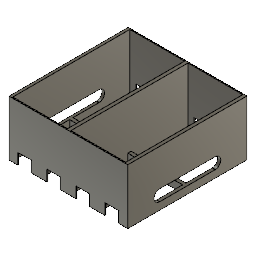
Jar Holder (Autodesk Fusion 360 design; units mm, degrees)
Autodesk Fusion 360 part; units mm, degrees
sketch "Schizzo1" plane through (0, 0, 0) normal (0, 0, 1) x (1, 0, 0)
  line L0 (0, 0) -> (214.4, 0)
  line L1 (214.4, 0) -> (214.4, 215)
  line L2 (214.4, 215) -> (0, 215)
  line L3 (0, 215) -> (0, 0)
  line L4 (51.4, 0) -> (5, 0)
  line L5 (57.4, 104.5) -> (103.8, 104.5)
  line L6 (57.4, 2) -> (57.4, 104.5)
  line L7 (103.8, 104.5) -> (103.8, 2)
  line L8 (109.8, 104.5) -> (156.2, 104.5)
  line L9 (109.8, 2) -> (109.8, 104.5)
  line L10 (156.2, 104.5) -> (156.2, 2)
  line L11 (162.2, 2) -> (162.2, 104.5)
  line L12 (162.2, 104.5) -> (208.6, 104.5)
  line L13 (208.6, 104.5) -> (208.6, 2)
  line L14 (5, 110.5) -> (5, 213)
  line L15 (5, 213) -> (51.4, 213)
  line L16 (51.4, 213) -> (51.4, 110.5)
  line L17 (57.4, 110.5) -> (57.4, 213)
  line L18 (57.4, 213) -> (103.8, 213)
  line L19 (103.8, 213) -> (103.8, 110.5)
  line L20 (109.8, 110.5) -> (109.8, 213)
  line L21 (109.8, 213) -> (156.2, 213)
  line L22 (156.2, 213) -> (156.2, 110.5)
  line L23 (162.2, 110.5) -> (162.2, 213)
  line L24 (162.2, 213) -> (208.6, 213)
  line L25 (208.6, 213) -> (208.6, 110.5)
  line L26 (5, 110.5) -> (51.4, 110.5)
  line L27 (103.8, 110.5) -> (57.4, 110.5)
  line L28 (109.8, 110.5) -> (156.2, 110.5)
  line L29 (208.6, 110.5) -> (162.2, 110.5)
  line L30 (57.4, 2) -> (103.8, 2)
  line L31 (156.2, 2) -> (109.8, 2)
  line L32 (162.2, 2) -> (208.6, 2)
  line L33 (5, 104.5) -> (51.4, 104.5)
  line L34 (51.4, 104.5) -> (51.4, 2)
  line L35 (51.4, 2) -> (5, 2)
  line L36 (5, 2) -> (5, 104.5)
  line L37 (5, 110.5) -> (5, 104.5)
  line L38 (51.4, 110.5) -> (51.4, 104.5)
  line L39 (51.4, 104.5) -> (57.4, 104.5)
  line L40 (51.4, 110.5) -> (57.4, 110.5)
  line L41 (103.8, 110.5) -> (109.8, 110.5)
  line L42 (103.8, 104.5) -> (109.8, 104.5)
  line L43 (103.8, 110.5) -> (103.8, 104.5)
  line L44 (109.8, 110.5) -> (109.8, 104.5)
  line L45 (57.4, 110.5) -> (57.4, 104.5)
  line L46 (156.2, 110.5) -> (156.2, 104.5)
  line L47 (162.2, 110.5) -> (162.2, 104.5)
  line L48 (156.2, 110.5) -> (162.2, 110.5)
  line L49 (156.2, 104.5) -> (5.3108, 104.5)
  line L50 (4.8606, 104.5) -> (-21.6126, 104.5)
  line L51 (-21.6126, 104.5) -> (-37.5505, 104.5)
  line L52 (5, 213) -> (5, 215)
  line L53 (5, 2) -> (5, 0)
  line L54 (208.6, 2) -> (208.6, 0)
  line L55 (162.2, 104.5) -> (156.2, 104.5)
  line L56 (208.6, 213) -> (208.6, 215)
  line L57 (208.6, 110.5) -> (208.6, 104.5)
  line L58 (80.6, 2) -> (80.6, 0)
  line L59 (133, 2) -> (133, 0)
  line L60 (80.6, 213) -> (80.6, 215)
  line L61 (133, 213) -> (133, 215)
  line L62 (5, 2) -> (0, 2)
  line L63 (51.4, 2) -> (57.4, 2)
  line L64 (103.8, 2) -> (109.8, 2)
  line L65 (156.2, 2) -> (162.2, 2)
  line L66 (208.6, 2) -> (214.4, 2)
  line L67 (208.6, 213) -> (214.4, 213)
  line L68 (156.2, 213) -> (162.2, 213)
  line L69 (103.8, 213) -> (109.8, 213)
  line L70 (51.4, 213) -> (57.4, 213)
  line L71 (0, 213) -> (5, 213)
  dimension "d1" = 214.4
  dimension "d2" = 215
  dimension "d6" = 46.4
  dimension "d7" = 102.5
  dimension "d8" = 46.4
  dimension "d9" = 102.5
  dimension "d10" = 46.4
  dimension "d11" = 102.5
  dimension "d13" = 6
  dimension "d14" = 6
  dimension "d15" = 46.4
  dimension "d16" = 102.5
  dimension "d17" = 46.4
  dimension "d19" = 46.4
  dimension "d20" = 102.5
  dimension "d21" = 46.4
  dimension "d22" = 102.5
  dimension "d23" = 6
  dimension "d24" = 6
  dimension "d25" = 6
  dimension "d26" = 46.4
  dimension "d27" = 102.5
  dimension "d28" = 6
  dimension "d29" = 6
  constraint horizontal L0
  constraint vertical L1
  constraint horizontal L2
  constraint vertical L3
  constraint coincident L0.start L3.end
  constraint horizontal L4
  constraint collinear L0 L4
  constraint horizontal L5
  constraint vertical L7
  constraint vertical L6
  constraint horizontal L8
  constraint vertical L10
  constraint vertical L9
  constraint horizontal L12
  constraint vertical L13
  constraint vertical L11
  constraint horizontal L15
  constraint vertical L16
  constraint vertical L14
  constraint horizontal L18
  constraint vertical L19
  constraint vertical L17
  constraint horizontal L21
  constraint vertical L22
  constraint vertical L20
  constraint horizontal L24
  constraint vertical L25
  constraint vertical L23
  constraint perpendicular L16 L26
  constraint perpendicular L17 L27
  constraint perpendicular L22 L28
  constraint perpendicular L23 L29
  constraint perpendicular L7 L30
  constraint perpendicular L9 L31
  constraint perpendicular L13 L32
  constraint horizontal L33
  constraint vertical L34
  constraint horizontal L35
  constraint vertical L36
  constraint perpendicular L33 L37
  constraint perpendicular L6 L39
  constraint perpendicular L17 L40
  constraint perpendicular L20 L41
  constraint perpendicular L9 L42
  constraint perpendicular L47 L48
  constraint perpendicular L14 L49
  constraint perpendicular L14 L50
  constraint perpendicular L14 L51
  constraint coincident L2 L52.end
  constraint perpendicular L2 L52
  constraint perpendicular L35 L53
  constraint coincident L0 L54.end
  constraint perpendicular L0 L54
  constraint perpendicular L46 L55
  constraint coincident L2 L56.end
  constraint perpendicular L2 L56
  constraint midpoint L30 L58.start
  constraint coincident L0 L58.end
  constraint perpendicular L0 L58
  constraint midpoint L31 L59.start
  constraint coincident L0 L59.end
  constraint perpendicular L0 L59
  constraint midpoint L18 L60.start
  constraint coincident L2 L60.end
  constraint perpendicular L2 L60
  constraint midpoint L21 L61.start
  constraint coincident L2 L61.end
  constraint perpendicular L2 L61
  constraint coincident L3 L62.end
  constraint perpendicular L3 L62
  constraint coincident L1 L66.end
  constraint perpendicular L1 L66
  constraint coincident L1 L67.end
  constraint perpendicular L1 L67
  constraint perpendicular L20 L69
  constraint coincident L3 L71.start
  constraint perpendicular L14 L71
  measures "d1" distance of L0.start L0.end
  measures "d2" distance of L0.start L2.end
  measures "d6" distance of L5.start L5.end
  measures "d7" distance of L6.start L5.start
  measures "d8" distance of L8.start L8.end
  measures "d9" distance of L8.start L9.start
  measures "d10" distance of L11.end L12.end
  measures "d11" distance of L11.end L11.start
  measures "d13" distance of L7 L9
  measures "d14" distance of L10 L11
  measures "d15" distance of L14.end L15.end
  measures "d16" distance of L14.start L14.end
  measures "d17" distance of L17.end L18.end
  measures "d19" distance of L20.end L21.end
  measures "d20" distance of L20.end L20.start
  measures "d21" distance of L23.end L24.end
  measures "d22" distance of L23.end L23.start
  measures "d23" distance of L16 L17
  measures "d24" distance of L19 L20
  measures "d25" distance of L22 L23
  measures "d26" distance of L33.start L33.end
  measures "d27" distance of L33.start L35.end
  measures "d28" distance of L6 L34
  measures "d29" distance of L26 L33
extrude "Estrusione1" add sketch "Schizzo1" along normal blind 100 contours L0 L3 L53 L62 | L0 L4 L30 L35 L53 L58 L63 | L3 L14 L36 L37 L62 L71 | L0 L30 L31 L58 L59 L64 | L6 L34 L39 L49 L63 | L26 L33 L37 L38 L49 | L2 L3 L52 L71 | L0 L31 L32 L54 L59 L65 | L38 L39 L40 L45 L49 | L2 L15 L18 L52 L60 L70 | L0 L1 L54 L66 | L7 L9 L42 L49 L64 | L16 L17 L40 L70 | L5 L27 L43 L45 L49 | L1 L13 L25 L57 L66 L67 | L10 L11 L55 L65 | L41 L42 L43 L44 L49 | L2 L18 L21 L60 L61 L69 | L12 L29 L47 L57 | L8 L28 L44 L46 L49 | L46 L47 L48 L55 | L19 L20 L41 L69 | L2 L21 L24 L56 L61 L68 | L1 L2 L56 L67 | L22 L23 L48 L68 makes body 1
sketch "Schizzo2" plane through (0, 0, 0) normal (0, 0, 1) x (1, 0, 0)
  line L0 (16, 222.0493) -> (40.4, 222.0493)
  line L1 (40.4, 222.0493) -> (40.4, 197.6493)
  line L2 (40.4, 197.6493) -> (16, 197.6493)
  line L3 (16, 197.6493) -> (16, 222.0493)
  line L4 (5, 110.5) -> (5, 213)
  line L5 (68.4, 222.0493) -> (92.8, 222.0493)
  line L6 (92.8, 222.0493) -> (92.8, 197.6493)
  line L7 (68.4, 197.6493) -> (68.4, 222.0493)
  line L8 (92.8, 197.6493) -> (68.4, 197.6493)
  line L9 (120.8, 197.6493) -> (120.8, 222.0493)
  line L10 (145.2, 197.6493) -> (120.8, 197.6493)
  line L11 (145.2, 222.0493) -> (145.2, 197.6493)
  line L12 (120.8, 222.0493) -> (145.2, 222.0493)
  line L13 (173.2, 222.0493) -> (197.6, 222.0493)
  line L14 (173.2, 197.6493) -> (173.2, 222.0493)
  line L15 (197.6, 197.6493) -> (173.2, 197.6493)
  line L16 (197.6, 222.0493) -> (197.6, 197.6493)
  line L17 (92.8, -12.3507) -> (68.4, -12.3507)
  line L18 (16, 12.0493) -> (40.4, 12.0493)
  line L19 (16, -12.3507) -> (16, 12.0493)
  line L20 (40.4, -12.3507) -> (16, -12.3507)
  line L21 (40.4, 12.0493) -> (40.4, -12.3507)
  line L22 (68.4, -12.3507) -> (68.4, 12.0493)
  line L23 (68.4, 12.0493) -> (92.8, 12.0493)
  line L24 (92.8, 12.0493) -> (92.8, -12.3507)
  line L25 (120.8, -12.3507) -> (120.8, 12.0493)
  line L26 (120.8, 12.0493) -> (145.2, 12.0493)
  line L27 (145.2, -12.3507) -> (120.8, -12.3507)
  line L28 (145.2, 12.0493) -> (145.2, -12.3507)
  line L29 (173.2, -12.3507) -> (173.2, 12.0493)
  line L30 (173.2, 12.0493) -> (197.6, 12.0493)
  line L31 (197.6, 12.0493) -> (197.6, -12.3507)
  line L32 (197.6, -12.3507) -> (173.2, -12.3507)
  dimension "d32" = 24.4
  dimension "d33" = 24.4
  dimension "d34" = 11
  dimension "d35" = 24.4
  dimension "d36" = 24.4
  dimension "d37" = 24.4
  dimension "d38" = 24.4
  dimension "d39" = 24.4
  dimension "d40" = 24.4
  dimension "d41" = 24.4
  dimension "d42" = 24.4
  dimension "d43" = 24.4
  dimension "d44" = 24.4
  dimension "d45" = 24.4
  dimension "d46" = 24.4
  dimension "d47" = 24.4
  dimension "d48" = 24.4
  constraint horizontal L0
  constraint vertical L1
  constraint horizontal L2
  constraint vertical L3
  constraint horizontal L5
  constraint vertical L6
  constraint horizontal L8
  constraint vertical L7
  constraint horizontal L12
  constraint vertical L11
  constraint horizontal L10
  constraint vertical L9
  constraint horizontal L13
  constraint vertical L16
  constraint horizontal L15
  constraint vertical L14
  constraint horizontal L18
  constraint vertical L21
  constraint horizontal L20
  constraint vertical L19
  constraint horizontal L23
  constraint vertical L24
  constraint horizontal L17
  constraint vertical L22
  constraint horizontal L26
  constraint vertical L28
  constraint horizontal L27
  constraint vertical L25
  constraint horizontal L30
  constraint vertical L31
  constraint horizontal L32
  constraint vertical L29
  measures "d32" distance of L0.start L0.end
  measures "d33" distance of L0.start L2.end
  measures "d34" distance of L3 L4
  measures "d35" distance of L5.start L5.end
  measures "d36" distance of L5.start L7.start
  measures "d37" distance of L9.end L11.start
  measures "d38" distance of L9.start L9.end
  measures "d39" distance of L13.end L13.start
  measures "d40" distance of L14.start L13.start
  measures "d41" distance of L18.start L18.end
  measures "d42" distance of L18.start L19.start
  measures "d43" distance of L22.end L23.end
  measures "d44" distance of L17.end L22.end
  measures "d45" distance of L26.end L25.end
  measures "d46" distance of L25.start L25.end
  measures "d47" distance of L30.end L29.end
  measures "d48" distance of L29.start L29.end
extrude "Estrusione2" cut sketch "Schizzo2" along normal blind 20 bodies 1
sketch "Schizzo3" plane through (214.4, 0, 0) normal (1, 0, 0) x (0, 1, 0)
  line L0 (0, 0) -> (215, 0)
  line L1 (215, 0) -> (215, 100)
  line L2 (215, 100) -> (0, 100)
  line L3 (0, 100) -> (0, 0)
  line L4 (107.5, 100) -> (107.5, 0)
  line L5 (0, 100) -> (107.5, 0)
  line L6 (107.5, 100) -> (0, 0)
  line L7 (107.5, 100) -> (215, 0)
  line L8 (215, 100) -> (107.5, 0)
  constraint midpoint L2 L4.start
  constraint midpoint L0 L4.end
  constraint coincident L2.end L3.start
  constraint coincident L0.start L3.end
  constraint coincident L0.end L1.start
  constraint coincident L1.end L2.start
extrude "Estrusione3" cut sketch "Schizzo3" against normal blind 240 contours L2 L5 L6 bodies 1
extrude "Estrusione4" cut sketch "Schizzo3" against normal blind 250 contours L2 L7 L8 bodies 1
sketch "Schizzo4" plane through (0, 0, 0) normal (0, -1, 0) x (1, 0, 0)
  line L0 (92.8, 20) -> (92.8, 0)
  line L1 (92.8, 0) -> (120.8, 0)
  line L2 (120.8, 0) -> (120.8, 20)
  line L3 (120.8, 20) -> (145.2, 20)
  line L4 (145.2, 20) -> (145.2, 0)
  line L5 (145.2, 0) -> (173.2, 0)
  line L6 (173.2, 0) -> (173.2, 20)
  line L7 (173.2, 20) -> (197.6, 20)
  line L8 (197.6, 20) -> (197.6, 0)
  line L9 (197.6, 0) -> (214.4, 0)
  line L10 (214.4, 0) -> (214.4, 100)
  line L11 (214.4, 100) -> (0, 100)
  line L12 (0, 100) -> (0, 0)
  line L13 (0, 0) -> (16, 0)
  line L14 (16, 0) -> (16, 20)
  line L15 (16, 20) -> (40.4, 20)
  line L16 (40.4, 20) -> (40.4, 0)
  line L17 (40.4, 0) -> (68.4, 0)
  line L18 (68.4, 0) -> (68.4, 20)
  line L19 (68.4, 20) -> (92.8, 20)
  line L20 (5.9183, 101.7944) -> (28.8885, 79.6123)
  line L21 (5.9183, 101.7944) -> (-27.1493, 101.7944) construction
  line L22 (28.8885, 79.6123) -> (50.3095, 101.7944)
  line L23 (50.3095, 101.7944) -> (5.9183, 101.7944)
  line L24 (28.2, 20) -> (28.2, 105.2887)
  line L25 (57.4, 98.1395, -2) -> (103.8, 98.1395, -2)
  line L26 (80.6, 20, -1) -> (80.6, 98.1395, -2)
  line L27 (109.8, 98.1395, -2) -> (156.2, 98.1395, -2)
  line L28 (133, 20, -1) -> (133, 98.1395, -2)
  line L29 (162.2, 98.1395, -2) -> (208.6, 98.1395, -2)
  line L30 (185.4, 20, 0) -> (185.4, 98.1395, -2)
  line L31 (101.9095, 101.7944) -> (57.5183, 101.7944)
  line L32 (57.5183, 101.7944) -> (80.4885, 79.6123)
  line L33 (80.4885, 79.6123) -> (101.9095, 101.7944)
  line L34 (154.4095, 101.7944) -> (110.0183, 101.7944)
  line L35 (110.0183, 101.7944) -> (132.9885, 79.6123)
  line L36 (132.9885, 79.6123) -> (154.4095, 101.7944)
  line L37 (206.8095, 101.7944) -> (162.4183, 101.7944)
  line L38 (162.4183, 101.7944) -> (185.3885, 79.6123)
  line L39 (185.3885, 79.6123) -> (206.8095, 101.7944)
  dimension "d55" = 44
  dimension "d56" = 31.9324
  dimension "d57" = 31.9324
  dimension "d58" = 31.9324
  dimension "d59" = 31.9324
  constraint horizontal L21
  constraint perpendicular L20 L22
  constraint parallel L21 L23
  constraint midpoint L15 L24.start
  constraint perpendicular L11 L24
  constraint perpendicular L32 L33
  constraint perpendicular L35 L36
  constraint perpendicular L38 L39
  measures "d55" angle of L20 L21
  measures "d56" distance of L20.start L20.end
  measures "d57" distance of L32.end L31.end
  measures "d58" distance of L34.end L35.end
  measures "d59" distance of L37.end L38.end
extrude "Estrusione5" cut sketch "Schizzo4" against normal blind 250 contours L11 L20 L22 L24 | L11 L20 L24 | L11 L32 L33 | L11 L35 L36 | L11 L38 L39 bodies 1
sketch "Schizzo5" plane through (214.4, 0, 0) normal (1, 0, 0) x (0, 1, 0)
  line L0 (22.1992, 7.0177) -> (85.594, 7.0177)
  line L1 (85.594, 7.0177) -> (53.8966, 37.6275)
  line L2 (53.8966, 37.6275) -> (22.1992, 7.0177)
  line L3 (161.8966, 37.6275) -> (130.1992, 7.0177)
  line L4 (193.594, 7.0177) -> (161.8966, 37.6275)
  line L5 (130.1992, 7.0177) -> (193.594, 7.0177)
  dimension "d64" = 44
  dimension "d65" = 44
  dimension "d66" = 44
  dimension "d67" = 44
  measures "d64" angle of L0 L2
  measures "d65" angle of L0 L1
  measures "d66" angle of L3 L5
  measures "d67" angle of L4 L5
extrude "Estrusione6" cut sketch "Schizzo5" against normal blind 300 bodies 1
sketch "Schizzo6" plane through (0, 0, 0) normal (0, -1, 0) x (1, 0, 0)
  line L0 (80.4885, 79.6123) -> (59.3764, 100)
  line L1 (59.3764, 100) -> (48.5767, 100)
  line L2 (48.5767, 100) -> (28.8885, 79.6123)
  line L3 (28.8885, 79.6123) -> (7.7764, 100)
  line L4 (7.7764, 100) -> (0, 100)
  line L5 (0, 100) -> (0, 0)
  line L6 (0, 0) -> (16, 0)
  line L7 (16, 0) -> (16, 20)
  line L8 (16, 20) -> (40.4, 20)
  line L9 (40.4, 20) -> (40.4, 0)
  line L10 (40.4, 0) -> (68.4, 0)
  line L11 (68.4, 0) -> (68.4, 20)
  line L12 (68.4, 20) -> (92.8, 20)
  line L13 (92.8, 20) -> (92.8, 0)
  line L14 (92.8, 0) -> (120.8, 0)
  line L15 (120.8, 0) -> (120.8, 20)
  line L16 (120.8, 20) -> (145.2, 20)
  line L17 (145.2, 20) -> (145.2, 0)
  line L18 (145.2, 0) -> (173.2, 0)
  line L19 (173.2, 0) -> (173.2, 20)
  line L20 (173.2, 20) -> (197.6, 20)
  line L21 (197.6, 20) -> (197.6, 0)
  line L22 (197.6, 0) -> (214.4, 0)
  line L23 (214.4, 0) -> (214.4, 100)
  line L24 (214.4, 100) -> (205.0767, 100)
  line L25 (205.0767, 100) -> (185.3885, 79.6123)
  line L26 (185.3885, 79.6123) -> (164.2764, 100)
  line L27 (164.2764, 100) -> (152.6767, 100)
  line L28 (152.6767, 100) -> (132.9885, 79.6123)
  line L29 (132.9885, 79.6123) -> (111.8764, 100)
  line L30 (111.8764, 100) -> (100.1767, 100)
  line L31 (100.1767, 100) -> (80.4885, 79.6123)
  line L32 (29.1963, 62.0362) -> (10.7719, 44.2439)
  line L33 (10.7719, 44.2439) -> (47.6208, 44.2439)
  line L34 (47.6208, 44.2439) -> (29.1963, 62.0362)
  line L35 (80.6774, 62.2474) -> (99.2519, 44.6118)
  line L36 (62.4042, 44.2997) -> (80.6774, 62.2474)
  line L37 (99.2519, 44.6118) -> (62.4042, 44.2997)
  line L38 (152.4208, 44.2439) -> (133.9963, 62.0362)
  line L39 (133.9963, 62.0362) -> (115.5719, 44.2439)
  line L40 (115.5719, 44.2439) -> (152.4208, 44.2439)
  line L41 (167.2042, 44.2997) -> (185.4774, 62.2474)
  line L42 (204.0519, 44.6118) -> (167.2042, 44.2997)
  line L43 (185.4774, 62.2474) -> (204.0519, 44.6118)
  dimension "d70" = 44
  dimension "d71" = 44
  dimension "d72" = 44
  dimension "d73" = 44
  constraint horizontal L33
  constraint horizontal L40
  measures "d70" angle of L32 L33
  measures "d71" angle of L33 L34
  measures "d72" angle of L39 L40
  measures "d73" angle of L38 L40
extrude "Estrusione7" cut sketch "Schizzo6" against normal blind 310 contours L32 L33 L34 | L35 L36 L37 | L38 L39 L40 | L41 L42 L43 bodies 1
extrude "Estrusione8" add sketch "Schizzo1" along normal blind 25 separate body contours L0 L3 L53 L62 | L0 L4 L30 L35 L53 L58 L63 | L3 L14 L36 L37 L62 L71 | L0 L30 L31 L58 L59 L64 | L6 L34 L39 L49 L63 | L26 L33 L37 L38 L49 | L2 L3 L52 L71 | L0 L31 L32 L54 L59 L65 | L38 L39 L40 L45 L49 | L2 L15 L18 L52 L60 L70 | L0 L1 L54 L66 | L7 L9 L42 L49 L64 | L16 L17 L40 L70 | L5 L27 L43 L45 L49 | L1 L13 L25 L57 L66 L67 | L10 L11 L55 L65 | L41 L42 L43 L44 L49 | L2 L18 L21 L60 L61 L69 | L12 L29 L47 L57 | L8 L28 L44 L46 L49 | L46 L47 L48 L55 | L19 L20 L41 L69 | L2 L21 L24 L56 L61 L68 | L1 L2 L56 L67 | L22 L23 L48 L68 makes body 2
extrude "Estrusione9" cut sketch "Schizzo2" along normal blind 20 bodies 2
sketch "Schizzo7" plane through (0, 0, 0) normal (0, 0, 1) x (1, 0, 0)
extrude "Estrusione10" add sketch "Schizzo1" along normal blind 100 separate body contours L5 L27 L43 L45 L49 | L41 L42 L43 L44 L49 | L8 L28 L44 L46 L49 makes body 3
extrude "Estrusione11" add sketch "Schizzo1" along normal blind 100 separate body contours L0 L3 L53 L62 | L3 L14 L36 L37 L62 L71 | L2 L3 L52 L71 makes body 4
extrude "Estrusione12" add sketch "Schizzo1" along normal blind 100 separate body contours L0 L1 L54 L66 | L1 L13 L25 L57 L66 L67 | L1 L2 L56 L67 makes body 5
extrude "Estrusione13" add sketch "Schizzo1" along normal blind 100 separate body contours L0 L3 L53 L62 | L0 L4 L30 L35 L53 L58 L63 | L3 L14 L36 L37 L62 L71 | L0 L30 L31 L58 L59 L64 | L2 L3 L52 L71 | L0 L31 L32 L54 L59 L65 | L2 L15 L18 L52 L60 L70 | L0 L1 L54 L66 | L7 L9 L42 L49 L64 | L1 L13 L25 L57 L66 L67 | L41 L42 L43 L44 L49 | L2 L18 L21 L60 L61 L69 | L19 L20 L41 L69 | L2 L21 L24 L56 L61 L68 | L1 L2 L56 L67 makes body 6
extrude "Estrusione14" cut sketch "Schizzo2" along normal blind 20 bodies 6
combine "Combina1" operation add target body 2 tool bodies 6
sketch "Schizzo8" plane through (214.4, 0, 0) normal (1, 0, 0) x (0, 1, 0)
  line L0 (0, 0) -> (215, 0)
  line L1 (215, 0) -> (215, 100)
  line L2 (215, 100) -> (0, 100)
  line L3 (0, 100) -> (0, 0)
  line L4 (107.5, 100) -> (107.5, 0)
  line L5 (57.5, 13.5316) -> (157.5, 13.5316)
  arc A0 (157.5, 13.5316) -> (157.5, 33.5316) centre (157.5, 23.5316) ccw
  line L6 (157.5, 33.5316) -> (57.5, 33.5316)
  arc A1 (57.5, 33.5316) -> (57.5, 13.5316) centre (57.5, 23.5316) ccw
  line L7 (57.5, 23.5316) -> (157.5, 23.5316) construction
  point P0 (107.5, 23.5316)
  dimension "d90" = 50
  dimension "d91" = 20
  constraint midpoint L2 L4.start
  constraint midpoint L0 L4.end
  constraint tangent L5 A0
  constraint tangent A0 L6
  constraint parallel L5 L6
  constraint tangent L6 A1
  constraint tangent L5 A1
  constraint perpendicular L4 L7
  constraint coincident L4 P0
  constraint midpoint L7 P0
  measures "d90" distance of A0.centre P0
  measures "d91" diameter of A0
extrude "Estrusione15" cut sketch "Schizzo8" against normal blind 500 contours L4 L5 L6 A1 | L4 L5 A0 L6 bodies 2
extrude "Estrusione16" add 1 faces at (107.8, 124.1667, 33.5316) along direction (0, 0, -1) blind 21 on bodies 2 bodies 2
extrude "Estrusione17" add 1 faces at (107.8, 157.5, 26.865) along direction (0, 1, 0) blind 10 on bodies 2 bodies 2
extrude "Estrusione18" add 1 faces at (107.8, 57.5, 26.865) along direction (0, -1, 0) blind 10 on bodies 2 bodies 2
hidden bodies 1 3 4 5
